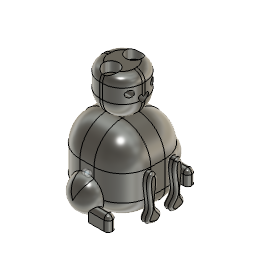
BUNNY BASE (Autodesk Fusion 360 design; units mm, degrees)
part number: 2026-03-05-09-03-59-716
Autodesk Fusion 360 part; units mm, degrees
note: some values were not read from the file. Chosen so that the rebuilt part matches the saved one: which face or edge a step refers to. Set by a fixed rule: which sketch regions a step uses.
sketch "Sketch1" plane through (0, 0, 0) normal (0, 0, 1) x (1, 0, 0)
  line L0 (0, 25) -> (0, 0)
  line L1 (0, 0) -> (25, 0)
  line L2 (25, 0) -> (25, 25)
  line L3 (25, 25) -> (0, 25)
  line L4 (35, 20) -> (50, 20)
  line L5 (50, 20) -> (50, 5)
  line L6 (50, 5) -> (35, 5)
  line L7 (35, 5) -> (35, 20)
  constraint coincident L0.end L1.start
  constraint vertical L0
  constraint perpendicular L0 L1
  constraint perpendicular L1 L2
  constraint perpendicular L0 L3
  constraint perpendicular L0 L4
  constraint perpendicular L4 L5
  constraint perpendicular L5 L6
  constraint perpendicular L4 L7
extrude "Extrude1" add sketch "Sketch1" along normal blind 25 contours L0 L1 L2 L3 makes body 1
extrude "Extrude2" add sketch "Sketch1" along normal blind 15 separate body contours L4 L5 L6 L7 makes body 2
fillet "Fillet1" radius 10 4 edges at (12.5, 25, 25) (25, 12.5, 25) (12.5, 0, 25) (0, 12.5, 25) on bodies 1
fillet "Fillet2" radius 3 4 edges at (42.5, 20, 15) (50, 12.5, 15) (42.5, 5, 15) (35, 12.5, 15) on bodies 2
fillet "Fillet3" radius 10 8 edges at (25, 0, 7.5) (22.0711, 2.9289, 22.0711) (0, 0, 7.5) (2.9289, 2.9289, 22.0711) (0, 25, 7.5) (2.9289, 22.0711, 22.0711) (25, 25, 7.5) (22.0711, 22.0711, 22.0711) on bodies 1
fillet "Fillet4" radius 7 8 edges at (50, 5, 6) (49.1213, 5.8787, 14.1213) (50, 20, 6) (49.1213, 19.1213, 14.1213) (35, 20, 6) (35.8787, 19.1213, 14.1213) (35, 5, 6) (35.8787, 5.8787, 14.1213) on bodies 2
fillet "Fillet5" radius 7 8 edges at (35, 12.5, 0) (37.0503, 7.0503, 0) (42.5, 5, 0) (47.9497, 7.0503, 0) (50, 12.5, 0) (47.9497, 17.9497, 0) (42.5, 20, 0) (37.0503, 17.9497, 0) on bodies 2
move_body "Move1" bodies 2 to x (1, 0, 0) y (0, 1, 0) z (0, 0, 1) at (-30, 0, 25)
fillet "Fillet6" radius 6 8 edges at (22.0711, 2.9289, 0) (25, 12.5, 0) (22.0711, 22.0711, 0) (12.5, 25, 0) (2.9289, 22.0711, 0) (0, 12.5, 0) (2.9289, 2.9289, 0) (12.5, 0, 0) on bodies 1
sketch "Sketch2" plane through (0, 0, 40) normal (0, 0, 1) x (-1, 0, 0)
  arc A0 (-8, -12) -> (-12, -8) centre (-12, -12) ccw
  line L0 (-12, -8) -> (-13, -8)
  arc A1 (-13, -8) -> (-17, -12) centre (-13, -12) ccw
  line L1 (-17, -12) -> (-17, -13)
  arc A2 (-17, -13) -> (-13, -17) centre (-13, -13) ccw
  line L2 (-13, -17) -> (-12, -17)
  arc A3 (-12, -17) -> (-8, -13) centre (-12, -13) ccw
  line L3 (-8, -13) -> (-8, -12)
  line L4 (-17, -12.5) -> (-8, -12.5) construction
  circle A4 centre (-12.5, -8.5) radius 2.75
  circle A5 centre (-12.5, -16.5) radius 2.75
  dimension "d17" = 5.5
  dimension "d18" = 5.5
  dimension "d19" = 4
  dimension "d20" = 4
  constraint midpoint L1 L4.start
  constraint midpoint L3 L4.end
  measures "d17" diameter of A4
  measures "d18" diameter of A5
  measures "d19" distance of L4 A5.centre
  measures "d20" distance of L4 A4.centre
extrude "Extrude3" cut sketch "Sketch2" against normal blind 3.5 contours A2 L2 A3 A5 | A2 L2 A3 A5 bodies 2
extrude "Extrude4" cut sketch "Sketch2" against normal blind 3.5 contours A0 L0 A1 A4 | A0 L0 A1 A4 bodies 2
sketch "Sketch3" plane through (0, 0, 25) normal (0, 0, 1) x (-1, 0, 0)
  line L0 (-10, -10) -> (-15, -10)
  line L1 (-15, -10) -> (-15, -15)
  line L2 (-15, -15) -> (-10, -15)
  line L3 (-10, -15) -> (-10, -10)
  line L4 (-12, -13) -> (-13, -13)
  line L5 (-13, -13) -> (-13, -12)
  line L6 (-13, -12) -> (-12, -12)
  line L7 (-12, -12) -> (-12, -13)
  constraint horizontal L4
  constraint perpendicular L4 L5
  constraint perpendicular L5 L6
  constraint perpendicular L4 L7
extrude "Extrude5" add sketch "Sketch3" against normal blind 1 contours L0 L1 L2 L3 | L4 L5 L6 L7 bodies 1 2
sketch "Sketch4" plane through (0, 0, 0) normal (-1, 0, 0) x (0, -1, 0)
  line L0 (-15, 6) -> (-10, 6)
  line L1 (-10, 6) -> (-10, 15)
  line L2 (-10, 15) -> (-15, 15)
  line L3 (-15, 15) -> (-15, 6)
  circle A0 centre (-12.5, 10.5) radius 2.75
  dimension "d27" = 5.5
  measures "d27" diameter of A0
extrude "Extrude6" cut sketch "Sketch4" against normal blind 3.5 contours L3 A0 | L1 L3 A0 | L1 A0 bodies 1
sketch "Sketch5" plane through (20, 0, 0) normal (1, 0, 0) x (0, 1, 0)
  line L0 (12, 32) -> (13, 32)
  line L1 (13, 32) -> (13, 37)
  line L2 (13, 37) -> (12, 37)
  line L3 (12, 37) -> (12, 32)
  circle A0 centre (16.5, 35) radius 1.118
  line L4 (12.5, 37) -> (12.5, 35.6537) construction
  circle A1 centre (8.5, 35) radius 1.118
  spline S0 degree 5 poles (12.5, 33) (12.5226, 33.0067) (12.5685, 33.025) (12.6399, 33.0668) (12.7396, 33.1472) (12.8718, 33.273) (13.0122, 33.4044) (13.1606, 33.5219) (13.3165, 33.609) (13.4777, 33.6559) (13.6407, 33.6591) (13.8008, 33.6201) (13.9522, 33.5435) (14.0883, 33.4359) (14.202, 33.304) (14.2858, 33.154) (14.3333, 32.9918) (14.3394, 32.8228) (14.3018, 32.6517) (14.2213, 32.4825) (14.1022, 32.3187) (13.9515, 32.1625) (13.7781, 32.0156) (13.5919, 31.8785) (13.4034, 31.751) (13.2228, 31.6314) (13.0593, 31.5174) (12.9198, 31.407) (12.8082, 31.2995) (12.7242, 31.1968) (12.6622, 31.1041) (12.6101, 31.032) (12.5527, 30.9924) (12.4765, 30.9949) (12.3746, 31.0421) (12.2491, 31.1275) (12.107, 31.2399) (11.9583, 31.3659) (11.8129, 31.4934) (11.6776, 31.615) (11.5544, 31.7294) (11.4428, 31.8396) (11.34, 31.9507) (11.2432, 32.0684) (11.1501, 32.1972) (11.0604, 32.3386) (10.9757, 32.4919) (10.899, 32.6546) (10.835, 32.823) (10.7895, 32.9927) (10.7696, 33.1591) (10.7824, 33.3177) (10.8335, 33.4636) (10.9248, 33.5921) (11.0537, 33.6979) (11.2103, 33.7755) (11.3801, 33.8196) (11.5474, 33.8264) (11.6979, 33.7941) (11.8224, 33.7241) (11.92, 33.6218) (11.9971, 33.4963) (12.0633, 33.3596) (12.1294, 33.2252) (12.204, 33.1076) (12.2905, 33.0215) (12.3694, 32.9875) (12.4332, 32.9849) (12.4774, 32.9933) (12.5, 33) knots 0 0 0 0 0 0 0.01538462 0.03076923 0.04615385 0.06153846 0.07692308 0.09230769 0.10769231 0.12307692 0.13846154 0.15384615 0.16923077 0.18461538 0.2 0.21538462 0.23076923 0.24615385 0.26153846 0.27692308 0.29230769 0.30769231 0.32307692 0.33846154 0.35384615 0.36923077 0.38461538 0.4 0.41538462 0.43076923 0.44615385 0.46153846 0.47692308 0.49230769 0.50769231 0.52307692 0.53846154 0.55384615 0.56923077 0.58461538 0.6 0.61538462 0.63076923 0.64615385 0.66153846 0.67692308 0.69230769 0.70769231 0.72307692 0.73846154 0.75384615 0.76923077 0.78461538 0.8 0.81538462 0.83076923 0.84615385 0.86153846 0.87692308 0.89230769 0.90769231 0.92307692 0.93846154 0.95384615 0.96923077 0.98461538 1 1 1 1 1 1
  point P0 (13.2116, 33.5453)
  point P1 (14, 33.5)
  point P2 (14.3147, 32.7349)
  point P3 (13.4593, 31.7894)
  point P4 (12.7164, 31.1816)
  point P5 (12.5, 31)
  point P6 (11.8609, 31.4517)
  point P7 (11.2531, 32.0595)
  point P8 (10.8254, 32.87)
  point P9 (10.9605, 33.6128)
  point P10 (11.7259, 33.7704)
  point P11 (12.1311, 33.2301)
  constraint midpoint L2 L4.start
  constraint perpendicular L2 L4
  constraint symmetric A0 L4 A1
extrude "Extrude7" cut sketch "Sketch5" against normal blind 3 contours L0 L1 L3 S0 | L0 L1 L3 S0 | A0 | A1 bodies 1
sketch "Sketch6" plane through (0, 0, 0) normal (0, -1, 0) x (1, 0, 0)
  line L0 (10, 6) -> (15, 6)
  line L1 (15, 6) -> (15, 15)
  line L2 (15, 15) -> (10, 15)
  line L3 (10, 15) -> (10, 6)
  circle A0 centre (12.5, 6) radius 5.9201
  constraint midpoint L0 A0.centre
extrude "Extrude8" add sketch "Sketch6" along normal blind 5 contours L0 L1 L3 A0 | L0 L1 L3 A0 bodies 1
sketch "Sketch7" plane through (0, 0, 0) normal (0, 0, 1) x (1, 0, 0)
  line L0 (0, 12) -> (1, 12)
  constraint horizontal L0
sketch "Sketch8" plane through (0, 25, 0) normal (0, 1, 0) x (-1, 0, 0)
  line L0 (-15, 6) -> (-10, 6)
  line L1 (-10, 6) -> (-10, 15)
  line L2 (-10, 15) -> (-15, 15)
  line L3 (-15, 15) -> (-15, 6)
  circle A0 centre (-12.5, 6) radius 5.92
  dimension "d34" = 11.84
  constraint midpoint L0 A0.centre
  measures "d34" diameter of A0
extrude "Extrude9" add sketch "Sketch8" along normal blind 5.92 contours L0 L1 L3 A0 | L0 L1 L3 A0 bodies 1
fillet "Fillet7" radius 5.9 1 edges at (6.9806, -5, 3.8592) on bodies 1
fillet "Fillet8" radius 5.9 1 edges at (18.0194, 30.92, 3.8592) on bodies 1
sketch "Sketch9" plane through (25, 0, 0) normal (1, 0, 0) x (0, 1, 0)
  line L0 (10, 6) -> (15, 6)
  line L1 (15, 6) -> (15, 15)
  line L2 (15, 15) -> (10, 15)
  line L3 (10, 15) -> (10, 6)
  line L4 (12.5, 6) -> (12.5, 15) construction
  spline S0 degree 5 poles (16, 15) (15.9219, 14.8926) (15.777, 14.6549) (15.5965, 14.2335) (15.4377, 13.5564) (15.3726, 12.563) (15.4207, 11.4714) (15.5494, 10.3319) (15.7185, 9.1929) (15.8852, 8.0984) (16.0094, 7.0845) (16.0582, 6.1767) (16.0114, 5.3865) (15.8617, 4.7131) (15.6149, 4.1458) (15.2898, 3.6653) (14.9182, 3.2465) (14.5453, 2.8599) (14.2281, 2.4747) (14.0218, 2.0663) (13.9691, 1.6239) (14.0878, 1.1574) (14.3596, 0.7043) (14.7453, 0.3141) (15.1981, 0.0324) (15.677, -0.1128) (16.1631, -0.1299) (16.6541, -0.0537) (17.1521, 0.0742) (17.6542, 0.219) (18.1398, 0.374) (18.57, 0.562) (18.9043, 0.8113) (19.1112, 1.1421) (19.1847, 1.5422) (19.146, 1.9676) (19.0281, 2.369) (18.8659, 2.7112) (18.6819, 2.9985) (18.4911, 3.2633) (18.3055, 3.5531) (18.142, 3.9154) (18.0208, 4.3902) (17.96, 5.0081) (17.9713, 5.7862) (18.0552, 6.7252) (18.1954, 7.8052) (18.3622, 8.9892) (18.5183, 10.2274) (18.624, 11.4621) (18.642, 12.6316) (18.5427, 13.6754) (18.3095, 14.5377) (17.9439, 15.1726) (17.4712, 15.5485) (16.9431, 15.6513) (16.5266, 15.5162) (16.2454, 15.2995) (16.0781, 15.1074) (16, 15) knots 0 0 0 0 0 0 0.018182 0.036364 0.054545 0.072727 0.090909 0.109091 0.127273 0.145455 0.163636 0.181818 0.2 0.218182 0.236364 0.254545 0.272727 0.290909 0.309091 0.327273 0.345455 0.363636 0.381818 0.4 0.418182 0.436364 0.454545 0.472727 0.490909 0.509091 0.527273 0.545455 0.563636 0.581818 0.6 0.618182 0.636364 0.654545 0.672727 0.690909 0.709091 0.727273 0.745455 0.763636 0.781818 0.8 0.818182 0.836364 0.854545 0.872727 0.890909 0.909091 0.927273 0.945455 0.963636 0.981818 1 1 1 1 1 1
  spline S1 degree 5 poles (9, 15) (9.0781, 14.8926) (9.223, 14.6549) (9.4035, 14.2335) (9.5623, 13.5564) (9.6274, 12.563) (9.5793, 11.4714) (9.4506, 10.3319) (9.2815, 9.1929) (9.1148, 8.0984) (8.9906, 7.0845) (8.9418, 6.1767) (8.9886, 5.3865) (9.1383, 4.7131) (9.3851, 4.1458) (9.7102, 3.6653) (10.0818, 3.2465) (10.4547, 2.8599) (10.7719, 2.4747) (10.9782, 2.0663) (11.0309, 1.6239) (10.9122, 1.1574) (10.6404, 0.7043) (10.2547, 0.3141) (9.8019, 0.0324) (9.323, -0.1128) (8.8369, -0.1299) (8.3459, -0.0537) (7.8479, 0.0742) (7.3458, 0.219) (6.8602, 0.374) (6.43, 0.562) (6.0957, 0.8113) (5.8888, 1.1421) (5.8153, 1.5422) (5.854, 1.9676) (5.9719, 2.369) (6.1341, 2.7112) (6.3181, 2.9985) (6.5089, 3.2633) (6.6945, 3.5531) (6.858, 3.9154) (6.9792, 4.3902) (7.04, 5.0081) (7.0287, 5.7862) (6.9448, 6.7252) (6.8046, 7.8052) (6.6378, 8.9892) (6.4817, 10.2274) (6.376, 11.4621) (6.358, 12.6316) (6.4573, 13.6754) (6.6905, 14.5377) (7.0561, 15.1726) (7.5288, 15.5485) (8.0569, 15.6513) (8.4734, 15.5162) (8.7546, 15.2995) (8.9219, 15.1074) (9, 15) knots 0 0 0 0 0 0 0.018182 0.036364 0.054545 0.072727 0.090909 0.109091 0.127273 0.145455 0.163636 0.181818 0.2 0.218182 0.236364 0.254545 0.272727 0.290909 0.309091 0.327273 0.345455 0.363636 0.381818 0.4 0.418182 0.436364 0.454545 0.472727 0.490909 0.509091 0.527273 0.545455 0.563636 0.581818 0.6 0.618182 0.636364 0.654545 0.672727 0.690909 0.709091 0.727273 0.745455 0.763636 0.781818 0.8 0.818182 0.836364 0.854545 0.872727 0.890909 0.909091 0.927273 0.945455 0.963636 0.981818 1 1 1 1 1 1
  line L5 (16.8286, 16.1404) -> (15.1714, 13.8596)
  line L6 (8.1714, 16.1404) -> (9.8286, 13.8596)
  point P0 (16, 7)
  point P1 (15, 3.3458)
  point P2 (14.0104, 1.6381)
  point P3 (15.3136, 0.0202)
  point P4 (17.4258, 0.1551)
  point P5 (19, 1)
  point P6 (18.9987, 2.4021)
  point P7 (18.4145, 3.3907)
  point P8 (18, 6)
  point P9 (18, 15)
  point P10 (9, 7)
  point P11 (10, 3.3458)
  point P12 (10.9896, 1.6381)
  point P13 (9.6864, 0.0202)
  point P14 (7.5742, 0.1551)
  point P15 (6, 1)
  point P16 (6.0013, 2.4021)
  point P17 (6.5855, 3.3907)
  point P18 (7, 6)
  point P19 (7, 15)
  constraint midpoint L0 L4.start
  constraint midpoint L2 L4.end
  constraint midpoint S0.start L5
  constraint symmetric L4 S0.start S1.start
  constraint symmetric L4 P0 P10
  constraint symmetric L4 P1 P11
  constraint symmetric L4 P2 P12
  constraint symmetric L4 P3 P13
  constraint symmetric L4 P4 P14
  constraint symmetric L4 P5 P15
  constraint symmetric L4 P6 P16
  constraint symmetric L4 P7 P17
  constraint symmetric L4 P8 P18
  constraint symmetric L4 P9 P19
  constraint symmetric L4 L5.start L6.start
  constraint symmetric L4 L5.end L6.end
extrude "Extrude10" add sketch "Sketch9" along normal blind 3 separate body contours S0 | S1 makes body 3 at (27.1186, 15.4112, 12.8892) makes body 4 at (27.1186, 9.5888, 12.8892)
fillet "Fillet9" radius 0.9 1 edges at (28, 17.8925, 0.2992) on bodies 3
fillet "Fillet10" radius 0.9 1 edges at (28, 7.1075, 0.2992) on bodies 4
fillet "Fillet11" radius 0.9 1 edges at (25, 17.8925, 0.2992) on bodies 3
fillet "Fillet12" radius 0.9 1 edges at (25, 7.1075, 0.2992) on bodies 4
sketch "Sketch10" plane through (0, 0, 0) normal (0, 0, 1) x (1, 0, 0)
  line L0 (16, 25) -> (23, 25)
  line L1 (23, 25) -> (23, 28)
  line L2 (23, 28) -> (16, 28)
  line L3 (16, 28) -> (16, 25)
  line L4 (0, 12) -> (1, 12)
  line L5 (16, 0) -> (16, -3)
  line L6 (23, 0) -> (23, -3)
  line L7 (16, -3) -> (23, -3)
  line L8 (16, 0) -> (23, 0)
  constraint horizontal L0
  constraint perpendicular L0 L1
  constraint perpendicular L1 L2
  constraint perpendicular L0 L3
  constraint perpendicular L6 L8
extrude "Extrude11" cut sketch "Sketch10" along normal blind 5 bodies 1
extrude "Extrude12" add sketch "Sketch10" along normal blind 5 bodies 1
fillet "Fillet13" radius 1.5 2 edges at (23, 0, 2.5) (23, -3, 2.5) on bodies 1
fillet "Fillet14" radius 1.5 2 edges at (23, 25, 2.5) (23, 28, 2.5) on bodies 1
fillet "Fillet15" radius 1.5 4 edges at (19.9175, 25, 5) (22.5607, 25.4393, 5) (22.5607, 27.5607, 5) (19.5067, 28, 5) on bodies 1
fillet "Fillet16" radius 1.5 5 edges at (19.9175, 0, 5) (22.5607, -0.4393, 5) (23, -1.5, 5) (19.2021, -3, 5) (22.5607, -2.5607, 5) on bodies 1
